Autodesk Inventor part; units mm, degrees
(part 2 of 2)
  spline S244 degree 2 poles (25.5687, -35.3765) (25.5292, -35.295) (25.3785, -35.216) (25.2476, -35.216) knots 0 0 0 1 2 2 2
  spline S245 degree 2 poles (25.2476, -35.216) (25.1241, -35.216) (24.8499, -35.3716) (24.7215, -35.4926) knots 0 0 0 1 2 2 2
  line L276 (24.7215, -35.4926) -> (24.7215, -37.2019)
  line L277 (24.7215, -37.2019) -> (24.3362, -37.2019)
  line L278 (24.3362, -37.2019) -> (24.3362, -34.9146)
  line L279 (24.3362, -34.9146) -> (24.7215, -34.9146)
  line L280 (24.7215, -34.9146) -> (24.7215, -35.1666)
  spline S246 degree 2 poles (24.7215, -35.1666) (24.8721, -35.0159) (25.1685, -34.8504) (25.3464, -34.8504) knots 0 0 0 1 2 2 2
  spline S247 degree 2 poles (25.3464, -34.8504) (25.5489, -34.8504) (25.8626, -35.0357) (25.9441, -35.2456) knots 0 0 0 1 2 2 2
  spline S248 degree 2 poles (25.9441, -35.2456) (26.1195, -35.0505) (26.4505, -34.8504) (26.6431, -34.8504) knots 0 0 0 1 2 2 2
  spline S249 degree 2 poles (26.6431, -34.8504) (26.7913, -34.8504) (27.0334, -34.9418) (27.1223, -35.0455) knots 0 0 0 1 2 2 2
  spline S250 degree 2 poles (27.1223, -35.0455) (27.2137, -35.1493) (27.315, -35.4605) (27.315, -35.6952) knots 0 0 0 1 2 2 2
  line L281 (27.315, -35.6952) -> (27.315, -37.2019)
  line L282 (27.315, -37.2019) -> (26.9297, -37.2019)
  spline S251 degree 2 poles (42.985, -37.271) (42.7578, -37.271) (42.3848, -37.1352) (42.2539, -37.0092) knots 0 0 0 1 2 2 2
  spline S252 degree 2 poles (42.2539, -37.0092) (42.1254, -36.8857) (41.9921, -36.5498) (41.9921, -36.3596) knots 0 0 0 1 2 2 2
  spline S253 degree 2 poles (41.9921, -36.3596) (41.9921, -36.1126) (42.2564, -35.6976) (42.5083, -35.5741) knots 0 0 0 1 2 2 2
  line L283 (42.5083, -35.5741) -> (42.5083, -35.5618)
  spline S254 degree 2 poles (42.5083, -35.5618) (42.2835, -35.4309) (42.0662, -35.1196) (42.0662, -34.8875) knots 0 0 0 1 2 2 2
  spline S255 degree 2 poles (42.0662, -34.8875) (42.0662, -34.5441) (42.5849, -34.0847) (42.985, -34.0847) knots 0 0 0 1 2 2 2
  spline S256 degree 2 poles (42.985, -34.0847) (43.4, -34.0847) (43.9014, -34.5194) (43.9014, -34.8603) knots 0 0 0 1 2 2 2
  spline S257 degree 2 poles (43.9014, -34.8603) (43.9014, -35.0653) (43.6618, -35.4654) (43.437, -35.5791) knots 0 0 0 1 2 2 2
  line L284 (43.437, -35.5791) -> (43.437, -35.5914)
  spline S258 degree 2 poles (43.437, -35.5914) (43.7038, -35.7149) (43.978, -36.0706) (43.978, -36.3522) knots 0 0 0 1 2 2 2
  spline S259 degree 2 poles (43.978, -36.3522) (43.978, -36.7424) (43.4098, -37.271) (42.985, -37.271) knots 0 0 0 1 2 2 2
  spline S260 degree 2 poles (43.558, -36.3917) (43.558, -36.204) (43.4098, -35.9817) (43.1999, -35.8681) knots 0 0 0 1 2 2 2
  spline S261 degree 2 poles (43.1999, -35.8681) (43.1307, -35.8285) (42.8986, -35.7371) (42.7528, -35.6779) knots 0 0 0 1 2 2 2
  spline S262 degree 2 poles (42.7528, -35.6779) (42.5849, -35.789) (42.4046, -36.12) (42.4046, -36.33) knots 0 0 0 1 2 2 2
  spline S263 degree 2 poles (42.4046, -36.33) (42.4046, -36.6066) (42.738, -36.9672) (42.9899, -36.9672) knots 0 0 0 1 2 2 2
  spline S264 degree 2 poles (42.9899, -36.9672) (43.2468, -36.9672) (43.558, -36.6585) (43.558, -36.3917) knots 0 0 0 1 2 2 2
  spline S265 degree 2 poles (43.5012, -34.8652) (43.5012, -34.6602) (43.2271, -34.386) (42.9825, -34.386) knots 0 0 0 1 2 2 2
  spline S266 degree 2 poles (42.9825, -34.386) (42.7602, -34.386) (42.4762, -34.6306) (42.4762, -34.8405) knots 0 0 0 1 2 2 2
  spline S267 degree 2 poles (42.4762, -34.8405) (42.4762, -34.9912) (42.6219, -35.2012) (42.7676, -35.2851) knots 0 0 0 1 2 2 2
  spline S268 degree 2 poles (42.7676, -35.2851) (42.8294, -35.3197) (43.0912, -35.4407) (43.1974, -35.4753) knots 0 0 0 1 2 2 2
  spline S269 degree 2 poles (43.1974, -35.4753) (43.3753, -35.3395) (43.5012, -35.0505) (43.5012, -34.8652) knots 0 0 0 1 2 2 2
  line L285 (48.3104, -37.2019) -> (48.3104, -35.8779)
  spline S270 degree 2 poles (48.3104, -35.8779) (48.3104, -35.7199) (48.2857, -35.4506) (48.2461, -35.3765) knots 0 0 0 1 2 2 2
  spline S271 degree 2 poles (48.2461, -35.3765) (48.2066, -35.295) (48.0559, -35.216) (47.925, -35.216) knots 0 0 0 1 2 2 2
  spline S272 degree 2 poles (47.925, -35.216) (47.8065, -35.216) (47.5348, -35.3617) (47.3915, -35.5) knots 0 0 0 1 2 2 2
  spline S273 degree 2 poles (47.3915, -35.5) (47.394, -35.5346) (47.3989, -35.6309) (47.3989, -35.6952) knots 0 0 0 1 2 2 2
  line L286 (47.3989, -35.6952) -> (47.3989, -37.2019)
  line L287 (47.3989, -37.2019) -> (47.0136, -37.2019)
  line L288 (47.0136, -37.2019) -> (47.0136, -35.8779)
  spline S274 degree 2 poles (47.0136, -35.8779) (47.0136, -35.7199) (46.9889, -35.4506) (46.9494, -35.3765) knots 0 0 0 1 2 2 2
  spline S275 degree 2 poles (46.9494, -35.3765) (46.9099, -35.295) (46.7592, -35.216) (46.6283, -35.216) knots 0 0 0 1 2 2 2
  spline S276 degree 2 poles (46.6283, -35.216) (46.5048, -35.216) (46.2306, -35.3716) (46.1022, -35.4926) knots 0 0 0 1 2 2 2
  line L289 (46.1022, -35.4926) -> (46.1022, -37.2019)
  line L290 (46.1022, -37.2019) -> (45.7168, -37.2019)
  line L291 (45.7168, -37.2019) -> (45.7168, -34.9146)
  line L292 (45.7168, -34.9146) -> (46.1022, -34.9146)
  line L293 (46.1022, -34.9146) -> (46.1022, -35.1666)
  spline S277 degree 2 poles (46.1022, -35.1666) (46.2528, -35.0159) (46.5492, -34.8504) (46.7271, -34.8504) knots 0 0 0 1 2 2 2
  spline S278 degree 2 poles (46.7271, -34.8504) (46.9296, -34.8504) (47.2433, -35.0357) (47.3248, -35.2456) knots 0 0 0 1 2 2 2
  spline S279 degree 2 poles (47.3248, -35.2456) (47.5002, -35.0505) (47.8312, -34.8504) (48.0238, -34.8504) knots 0 0 0 1 2 2 2
  spline S280 degree 2 poles (48.0238, -34.8504) (48.172, -34.8504) (48.4141, -34.9418) (48.503, -35.0455) knots 0 0 0 1 2 2 2
  spline S281 degree 2 poles (48.503, -35.0455) (48.5944, -35.1493) (48.6957, -35.4605) (48.6957, -35.6952) knots 0 0 0 1 2 2 2
  line L294 (48.6957, -35.6952) -> (48.6957, -37.2019)
  line L295 (48.6957, -37.2019) -> (48.3104, -37.2019)
  line L296 (51.8301, -37.2019) -> (51.8301, -35.8779)
  spline S282 degree 2 poles (51.8301, -35.8779) (51.8301, -35.7199) (51.8054, -35.4506) (51.7659, -35.3765) knots 0 0 0 1 2 2 2
  spline S283 degree 2 poles (51.7659, -35.3765) (51.7264, -35.295) (51.5757, -35.216) (51.4448, -35.216) knots 0 0 0 1 2 2 2
  spline S284 degree 2 poles (51.4448, -35.216) (51.3263, -35.216) (51.0545, -35.3617) (50.9113, -35.5) knots 0 0 0 1 2 2 2
  spline S285 degree 2 poles (50.9113, -35.5) (50.9138, -35.5346) (50.9187, -35.6309) (50.9187, -35.6952) knots 0 0 0 1 2 2 2
  line L297 (50.9187, -35.6952) -> (50.9187, -37.2019)
  line L298 (50.9187, -37.2019) -> (50.5334, -37.2019)
  line L299 (50.5334, -37.2019) -> (50.5334, -35.8779)
  spline S286 degree 2 poles (50.5334, -35.8779) (50.5334, -35.7199) (50.5087, -35.4506) (50.4692, -35.3765) knots 0 0 0 1 2 2 2
  spline S287 degree 2 poles (50.4692, -35.3765) (50.4296, -35.295) (50.279, -35.216) (50.1481, -35.216) knots 0 0 0 1 2 2 2
  spline S288 degree 2 poles (50.1481, -35.216) (50.0246, -35.216) (49.7504, -35.3716) (49.6219, -35.4926) knots 0 0 0 1 2 2 2
  line L300 (49.6219, -35.4926) -> (49.6219, -37.2019)
  line L301 (49.6219, -37.2019) -> (49.2366, -37.2019)
  line L302 (49.2366, -37.2019) -> (49.2366, -34.9146)
  line L303 (49.2366, -34.9146) -> (49.6219, -34.9146)
  line L304 (49.6219, -34.9146) -> (49.6219, -35.1666)
  spline S289 degree 2 poles (49.6219, -35.1666) (49.7726, -35.0159) (50.069, -34.8504) (50.2469, -34.8504) knots 0 0 0 1 2 2 2
  spline S290 degree 2 poles (50.2469, -34.8504) (50.4494, -34.8504) (50.7631, -35.0357) (50.8446, -35.2456) knots 0 0 0 1 2 2 2
  spline S291 degree 2 poles (50.8446, -35.2456) (51.02, -35.0505) (51.351, -34.8504) (51.5436, -34.8504) knots 0 0 0 1 2 2 2
  spline S292 degree 2 poles (51.5436, -34.8504) (51.6918, -34.8504) (51.9339, -34.9418) (52.0228, -35.0455) knots 0 0 0 1 2 2 2
  spline S293 degree 2 poles (52.0228, -35.0455) (52.1142, -35.1493) (52.2155, -35.4605) (52.2155, -35.6952) knots 0 0 0 1 2 2 2
  line L305 (52.2155, -35.6952) -> (52.2155, -37.2019)
  line L306 (52.2155, -37.2019) -> (51.8301, -37.2019)
  point P0 (0, 0)
  dimension "d45" = 8.7721
  dimension "d46" = 40.64
  constraints: 18 end point, 17 horizontal
  measures "d45" distance between parallel lines of L1 L0
  measures "d46" distance between parallel lines of L6 L0
extrude "Extrusion4" cut sketch "Sketch7" against normal blind 1.5875
fillet "Fillet1" radius 1.5875 9 edges at (-55.626, 0, -12.7) (-30.48, 0, -12.7) (-1.651, 0, -12.7) (29.083, 0, -12.7) (38.9043, 0, 19.05) (13.7499, 0, 19.05) (-9.3726, 0, 19.05) (-32.4951, 0, 19.05) (-55.6175, 0, 19.05)
fillet "Fillet2" radius 1.5875 4 edges at (-63.5, -3.175, 44.45) (63.5, -3.175, 44.45) (63.5, -3.175, -44.45) (-63.5, -3.175, -44.45)
equation "\"gap0\" = frontGapBetweenHoles"
equation "\"gap1\" = 0.5 * hex5mmHole + 0.5 * hex4mmHole + frontGapBetweenHoles"
equation "\"gap2\" = 0.5 * hex6mmHole + 0.5 * hex5mmHole + frontGapBetweenHoles"
equation "\"gap3\" = 0.5 * hex7mmHole + 0.5 * hex6mmHole + frontGapBetweenHoles"
equation "\"gap4\" = 0.5 * hex8mmHole + 0.5 * hex7mmHole + frontGapBetweenHoles"
equation "\"gap5\" = backGapBetweenHoles"
equation "\"gap6\" = 0.5 * hex12mmHole + 0.5 * hex10mmHole + backGapBetweenHoles"
equation "\"gap7\" = 0.5 * hex14mmHole + 0.5 * hex12mmHole + backGapBetweenHoles"
equation "\"gap8\" = 0.5 * hex17mmHole + 0.5 * hex14mmHole + backGapBetweenHoles"
equation "\"d46\" = centerLineForBackText"
equation "\"frontGapBetweenHoles\" = 7.88247"
equation "\"backGapBetweenHoles\" = 7.874"
equation "\"centerLineForFrontText\" = 8.3185"
equation "\"centerLineForBackText\" = 40.64"
body "Solid1"
